skadis_nut_left (Autodesk Fusion 360 design; units mm, degrees)
part number: 2026-09-06-14-40-21-794
Autodesk Fusion 360 part; units mm, degrees
sketch "Plate" plane through (0, 0, 0) normal (0, 1, 0) x (1, 0, 0)
  line L0 (0, 0) -> (11, 0)
  line L1 (11, 0) -> (11, -48)
  line L2 (11, -48) -> (0, -48)
  line L3 (0, -48) -> (0, 0)
  dimension "d382" = 11
  dimension "d383" = 48
  constraint coincident L0.start L3.end
  constraint horizontal L0
  constraint horizontal L2
  constraint vertical L1
  constraint vertical L3
  measures "d382" horizontal distance of L0.start L1.end
  measures "d383" vertical distance of L0.start L1.end
extrude "Plate (1)" add sketch "Plate" along normal mid plane 33 from surface at 4.5
sketch "Hook profile" plane through (0, 0, 0) normal (0, 1, 0) x (1, 0, 0)
  line L0 (0, -46) -> (-8.3, -46)
  line L1 (-8.3, -46) -> (-8.3, -29)
  line L2 (-8.3, -29) -> (-5.3, -29)
  line L3 (-5.3, -29) -> (-3.8, -30.5)
  line L4 (-3.8, -30.5) -> (-3.8, -41)
  line L5 (-3.8, -41) -> (0, -41)
  line L6 (0, -41) -> (0, -46)
  dimension "d387" = 46
  dimension "d388" = 8.3
  dimension "d389" = 3.8
  dimension "d390" = 5
  dimension "d391" = 10.5
  dimension "d392" = 1.5
  dimension "d393" = 1.5
  constraint horizontal L0
  constraint horizontal L2
  constraint horizontal L5
  constraint vertical L1
  constraint vertical L4
  constraint vertical L6
  constraint coincident origin L6
  measures "d387" vertical distance of origin L0.start
  measures "d388" horizontal distance of L0.start L0.end
  measures "d389" horizontal distance of L4.end L5.end
  measures "d390" vertical distance of L0.start L5.end
  measures "d391" vertical distance of L3.end L4.end
  measures "d392" horizontal distance of L2.end L3.end
  measures "d393" vertical distance of L2.end L3.end
extrude "Hook profile (1)" add sketch "Hook profile" along normal mid plane 2.4
pattern_linear "Hook rows" count 2 spacing 25.4 along (0, 0, -1) count 3 spacing 0 along (0, 0, 1) of "Hook profile (1)"
sketch "Screw hole" plane through (0, 0, 0) normal (0, 1, 0) x (1, 0, 0)
  line L0 (-1, -21.6) -> (12, -21.6)
  line L1 (12, -21.6) -> (12, -26.4)
  line L2 (12, -26.4) -> (-1, -26.4)
  line L3 (-1, -26.4) -> (-1, -21.6)
  dimension "d400" = 12
  dimension "d401" = 21.6
  dimension "d402" = 13
  dimension "d403" = 4.8
  constraint horizontal L0
  constraint horizontal L2
  constraint vertical L1
  constraint vertical L3
  measures "d400" horizontal distance of origin L0.end
  measures "d401" vertical distance of origin L0.end
  measures "d402" horizontal distance of L0.start L0.end
  measures "d403" vertical distance of L0.end L1.end
extrude "Screw hole (1)" cut sketch "Screw hole" along normal mid plane 16.8 from surface at 7.52
sketch "Nut cavity" plane through (0, 0, 0) normal (0, 1, 0) x (1, 0, 0)
  line L0 (3.6, -20.3) -> (7, -20.3)
  line L1 (7, -20.3) -> (7, -27.7)
  line L2 (7, -27.7) -> (3.6, -27.7)
  line L3 (3.6, -27.7) -> (3.6, -20.3)
  dimension "d407" = 7
  dimension "d408" = 20.3
  dimension "d409" = 3.4
  dimension "d410" = 7.4
  constraint horizontal L0
  constraint horizontal L2
  constraint vertical L1
  constraint vertical L3
  measures "d407" horizontal distance of origin L0.end
  measures "d408" vertical distance of origin L0.end
  measures "d409" horizontal distance of L0.start L0.end
  measures "d410" vertical distance of L0.end L1.end
extrude "Nut cavity (1)" cut sketch "Nut cavity" along normal mid plane 19.4 from surface at 7.52
sketch "Nut entry" plane through (0, 0, 0) normal (0, 1, 0) x (1, 0, 0)
  line L0 (3.6, -26.7) -> (7, -26.7)
  line L1 (7, -26.7) -> (7, -49)
  line L2 (7, -49) -> (3.6, -49)
  line L3 (3.6, -49) -> (3.6, -26.7)
  dimension "d414" = 7
  dimension "d415" = 26.7
  dimension "d416" = 3.4
  dimension "d417" = 22.3
  constraint horizontal L0
  constraint horizontal L2
  constraint vertical L1
  constraint vertical L3
  measures "d414" horizontal distance of origin L0.end
  measures "d415" vertical distance of origin L0.end
  measures "d416" horizontal distance of L0.start L0.end
  measures "d417" vertical distance of L0.end L1.end
extrude "Nut entry (1)" cut sketch "Nut entry" along normal mid plane 7.4 from surface at 1.52
sketch "Cavity roof" plane through (0, 0, 0) normal (0, 0, 1) x (1, 0, 0)
  line L0 (3.6, -2.18) -> (7, -2.18)
  line L1 (7, -2.18) -> (5.3, -3.88)
  line L2 (5.3, -3.88) -> (3.6, -2.18)
  dimension "d421" = 3.6
  dimension "d422" = 2.18
  dimension "d423" = 7
  dimension "d424" = 5.3
  dimension "d425" = 1.7
  constraint horizontal L0
  measures "d421" horizontal distance of origin L0.start
  measures "d422" vertical distance of origin L0.start
  measures "d423" horizontal distance of origin L0.end
  measures "d424" horizontal distance of origin L1.end
  measures "d425" vertical distance of L0.start L1.end
extrude "Cavity roof (1)" cut sketch "Cavity roof" along normal mid plane 29.7 from surface at 34.15
equation "bracketWidth = 24.0 mm" comment "bracket width across the upright"
equation "plateHeight = 48.0 mm" comment "plate height"
equation "plateInboardExtension = 9.0 mm" comment "extra plate toward the desk centre, where the channel reaches"
equation "boardThickness = 6.0 mm" comment "measured SKADIS panel thickness"
equation "screwLength = 15.0 mm" comment "measured decorative M4 screw"
equation "screwDiameter = 4.0 mm" comment "M4 shank"
equation "screwClearance = 0.8 mm" comment "slack around the shank"
equation "screwTipClearance = 2.0 mm" comment "tip stops this short of the plate's back face"
equation "screwSlotWidth = screwDiameter + screwClearance" comment "screw relief slot height"
equation "nutAcrossFlats = 7.0 mm" comment "M4 square nut across flats"
equation "nutThickness = 3.0 mm" comment "M4 square nut thickness"
equation "nutChannelClearance = 0.4 mm" comment "slack around the nut in its channel"
equation "nutChannelHeight = nutAcrossFlats + nutChannelClearance" comment "channel height; under the nut's diagonal so it cannot turn"
equation "plateThickness = screwLength - boardThickness + screwTipClearance" comment "derived: deep enough to swallow the screw"
equation "mountTravel = 12.0 mm" comment "left-right adjustment"
equation "nutChannelLength = mountTravel + nutAcrossFlats + nutChannelClearance" comment "channel length along the plate"
equation "screwSlotLength = mountTravel + screwSlotWidth" comment "relief slot length along the plate"
equation "topMountZ = 24.0 mm" comment "top channel centre"
equation "mountOffsetY = 7.52 mm" comment "channel centre on the board's grid"
equation "slotOvershoot = 1.0 mm" comment "cuts reach past the faces they cut"
equation "slotWidth = 3.2 mm" comment "measured upright slot width"
equation "slotPitchVertical = 25.4 mm" comment "1 inch, measured"
equation "faceMetalThickness = 2.0 mm" comment "upright face metal"
equation "hookTabWidth = slotWidth - 0.8 mm" comment "blade width through the slot"
equation "hookThroat = faceMetalThickness + 1.8 mm" comment "gap behind the plate"
equation "hookNeckHeight = 5.0 mm" comment "bears on the slot bottom edge"
equation "hookLipThickness = 4.5 mm" comment "lip behind the upright face"
equation "hookLipDrop = 12.0 mm" comment "engagement below the neck"
equation "hookLipChamfer = 1.5 mm" comment "lead-in past slot burrs"
equation "topHookNeckTop = plateHeight - 2 mm" comment "top hook row"
equation "hookRows = 2" comment "hook rows (pattern count)"
equation "nutCavityClearance = 0.4 mm" comment "slack across the nut's thickness"
equation "nutWallThickness = 4.0 mm" comment "wall in front of the nut; the screw pulls the nut against it"
equation "nutCavityDepth = nutThickness + nutCavityClearance" comment "cavity depth"
equation "nutRoofDepth = nutCavityDepth / 2" comment "45 deg roof beyond the cavity's outboard end, so it prints unsupported"
equation "d382 = plateThickness"
equation "d383 = plateHeight"
equation "d384 = plateInboardExtension / 2"
equation "d385 = bracketWidth + plateInboardExtension"
equation "d387 = topHookNeckTop"
equation "d388 = hookThroat + hookLipThickness"
equation "d389 = hookThroat"
equation "d390 = hookNeckHeight"
equation "d391 = hookLipDrop - hookLipChamfer"
equation "d392 = hookLipChamfer"
equation "d393 = hookLipChamfer"
equation "d394 = hookTabWidth"
equation "d396 = hookRows"
equation "d398 = -slotPitchVertical"
equation "d400 = plateThickness + slotOvershoot"
equation "d401 = topMountZ - screwSlotWidth / 2"
equation "d402 = plateThickness + 2 * slotOvershoot"
equation "d403 = screwSlotWidth"
equation "d404 = mountOffsetY"
equation "d405 = screwSlotLength"
equation "d407 = plateThickness - nutWallThickness"
equation "d408 = topMountZ - nutChannelHeight / 2"
equation "d409 = nutCavityDepth"
equation "d410 = nutChannelHeight"
equation "d411 = mountOffsetY"
equation "d412 = nutChannelLength"
equation "d414 = plateThickness - nutWallThickness"
equation "d415 = topMountZ + nutChannelHeight / 2 - slotOvershoot"
equation "d416 = nutCavityDepth"
equation "d417 = plateHeight - topMountZ - nutChannelHeight / 2 + 2 * slotOvershoot"
equation "d418 = mountOffsetY - mountTravel / 2"
equation "d419 = nutChannelHeight"
equation "d421 = plateThickness - nutWallThickness - nutCavityDepth"
equation "d422 = -( mountOffsetY - nutChannelLength / 2 )"
equation "d423 = plateThickness - nutWallThickness"
equation "d424 = plateThickness - nutWallThickness - nutCavityDepth / 2"
equation "d425 = nutRoofDepth"
equation "d426 = ( topMountZ - nutChannelHeight / 2 + plateHeight ) / 2"
equation "d427 = plateHeight - topMountZ + nutChannelHeight / 2 + 2 * slotOvershoot"
named bodies: "skadis_nut_left"
